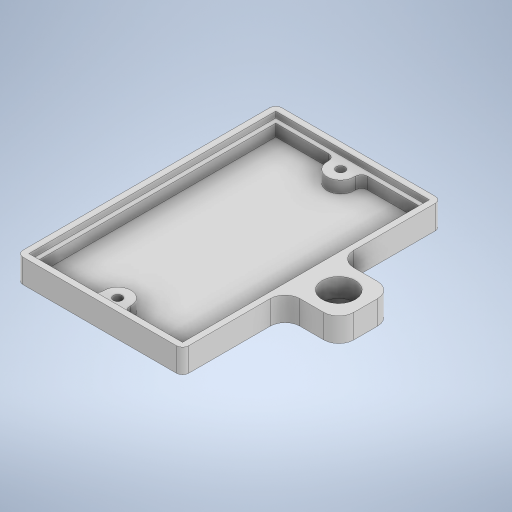
# Autodesk Inventor part: PermaProtoBase_HalfSizeScrewMount
Saved by Autodesk Inventor 2023 (Build 270158000, 158)
## iProperties
Created: 2023-02-17
Part Number: PermaProtoBase_HalfSizeScrewMount
Material: Generic
Document SubType Name: Modeling
Designer: User
Density: 1 g/cm^3
Appearance: Default
Author: User
Autodesk Inventor part; units mm, degrees
ref_plane "YZ Plane" through (0, 0, 0) normal (1, 0, 0) x (0, 1, 0)
ref_plane "XZ Plane" through (0, 0, 0) normal (0, 1, 0) x (-1, 0, 0)
ref_plane "XY Plane" through (0, 0, 0) normal (0, 0, 1) x (1, 0, 0)
sketch "Sketch1" plane through (0, 0, 0) normal (0, 1, 0) x (-1, 0, 0)
  line L0 (-27.75, 43.375) -> (27.75, 43.375)
  line L1 (27.75, 43.375) -> (27.75, -43.375)
  line L2 (27.75, -43.375) -> (-27.75, -43.375)
  line L3 (-27.75, -43.375) -> (-27.75, 43.375)
  line L4 (-27.75, 43.375) -> (27.75, -43.375) construction
  line L5 (27.75, 43.375) -> (-27.75, -43.375) construction
  point P0 (0, 0)
  dimension "d0" = 86.75
  dimension "d1" = 55.5
  constraints: 12 end point, 2 midpoint, 2 parallel, 1 horizontal, 1 perpendicular
  measures "d0" distance of L0.end L1.end
  measures "d1" distance of L1.end L2.end
extrude "Extrusion1" add sketch "Sketch1" along normal blind 8
sketch "Sketch2" plane through (0, 8, 0) normal (0, 1, 0) x (1, 0, 0)
  line L0 (25.75, -41.375) -> (-25.75, -41.375)
  line L1 (-25.75, -41.375) -> (-25.75, 41.375)
  line L2 (-25.75, 41.375) -> (25.75, 41.375)
  line L3 (25.75, 41.375) -> (25.75, -41.375)
  line L4 (25.75, -41.375) -> (-25.75, 41.375) construction
  line L5 (-25.75, -41.375) -> (25.75, 41.375) construction
  point P0 (0, 0)
  dimension "d4" = 51.5
  dimension "d5" = 82.75
  constraints: 12 end point, 2 midpoint, 2 parallel, 1 horizontal, 1 perpendicular
  measures "d4" distance of L1.end L2.end
  measures "d5" distance of L0.end L1.end
extrude "Extrusion2" cut sketch "Sketch2" against normal blind 2
sketch "Sketch3" plane through (0, 6, 0) normal (0, 1, 0) x (1, 0, 0)
  line L0 (24.25, 39.875) -> (-24.25, 39.875)
  line L1 (-24.25, 39.875) -> (-24.25, -39.875)
  line L2 (-24.25, -39.875) -> (24.25, -39.875)
  line L3 (24.25, -39.875) -> (24.25, 39.875)
  line L4 (24.25, 39.875) -> (-24.25, -39.875) construction
  line L5 (-24.25, 39.875) -> (24.25, -39.875) construction
  point P0 (0, 0)
  dimension "d8" = 79.75
  dimension "d9" = 48.5
  constraints: 12 end point, 2 midpoint, 2 parallel, 1 horizontal, 1 perpendicular
  measures "d8" distance of L0.end L1.end
  measures "d9" distance of L0.start L0.end
extrude "Extrusion3" cut sketch "Sketch3" against normal blind 4
sketch "Sketch4" plane through (0, 2, 0) normal (0, 1, 0) x (1, 0, 0)
  circle A0 centre (0, -37.375) radius 4.5
  circle A1 centre (0, 37.375) radius 4.5
  line L0 (24.25, -39.875) -> (-24.25, -39.875) projected
  line L1 (25.75, -41.375) -> (-25.75, -41.375) projected
  circle A2 centre (0, -37.375) radius 1.5
  circle A3 centre (0, 37.375) radius 1.5
  point P0 (0, 0)
  point P1 (-3.7417, -39.875)
  point P2 (3.7417, -39.875)
  dimension "d12" = 9
  dimension "d13" = 9
  dimension "d14" = 74.75
  dimension "d16" = 4
  dimension "d17" = 3
  dimension "d18" = 3
  constraints: 4 centre point, 2 coincident
  measures "d12" diameter of A0
  measures "d13" diameter of A1
  measures "d14" distance of A1.centre A0.centre
  measures "d16" distance from line of L1 A0.centre
  measures "d17" diameter of A2
  measures "d18" diameter of A3
extrude "Extrusion4" add sketch "Sketch4" along normal blind 4 contours A0 L0 | A1
sketch "Sketch5" plane through (27.75, 0, 43.375) normal (1, 0, 0) x (0, 0, -1)
  line L0 (84.75, 8) -> (2, 8) projected
  line L1 (0, 0) -> (86.75, 0) projected
  line L2 (34.375, 8) -> (52.375, 8)
  line L3 (52.375, 8) -> (52.375, 0)
  line L4 (52.375, 0) -> (34.375, 0)
  line L5 (34.375, 0) -> (34.375, 8)
  point P0 (43.375, 0)
  point P1 (34.375, 4)
  point P2 (43.375, 0)
  point P3 (34.375, 0)
  point P4 (52.375, 8)
  dimension "d21" = 18
  dimension "d22" = 9
  constraints: 8 end point, 2 midpoint, 2 parallel, 2 point on line, 1 horizontal, 1 perpendicular
  measures "d21" distance from line of point (34.375, 4) L3
  measures "d22" distance from line of point (43.375, 0) L3
extrude "Extrusion5" add sketch "Sketch5" along normal blind 18
sketch "Sketch6" plane through (0, 8, 0) normal (0, 1, 0) x (1, 0, 0)
  line L0 (27.75, -43.375) -> (27.75, -9) projected
  line L1 (27.75, -9) -> (45.75, -9) projected
  point P0 (0, 0)
  point P1 (36.75, 0)
  dimension "d32" = 9
  dimension "d33" = 9
  measures "d32" distance from line of L0 point (36.75, 0)
  measures "d33" distance from line of L1 point (36.75, 0)
hole "Hole1" at (36.75, 8, 0) direction (0, -1, 0) diameter 7.1437 end through all counterbore diameter 11.1125 counterbore depth 6.35
fillet "Fillet1" radius 2 8 edges at (3.7417, 4, -39.875) (-3.7417, 4, -39.875) (3.7417, 4, 39.875) (-3.7417, 4, 39.875) (27.75, 4, 43.375) (-27.75, 4, 43.375) (-27.75, 4, -43.375) (27.75, 4, -43.375)
fillet "Fillet2" radius 5 4 edges at (27.75, 4, 9) (45.75, 4, 9) (45.75, 4, -9) (27.75, 4, -9)
equation "\"d22\" = 0.5 * d21"
body "Solid1"
